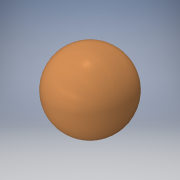
# Autodesk Inventor part: Ball
Saved by Autodesk Inventor 2016 (Build 200138000, 138)
## iProperties
Created: 2016-01-18
Part Number: Ball
Material: Polyurethane Foam
Document SubType Name: Modeling
Designer: yash
Density: 0.032 g/cm^3
Appearance: Coarse Textured - Umber
Author: yash
Autodesk Inventor part; units mm, degrees
ref_plane "YZ Plane" through (0, 0, 0) normal (1, 0, 0) x (0, 1, 0)
ref_plane "XZ Plane" through (0, 0, 0) normal (0, 1, 0) x (-1, 0, 0)
ref_plane "XY Plane" through (0, 0, 0) normal (0, 0, 1) x (1, 0, 0)
sketch "Sketch1" plane through (0, 0, 0) normal (0, 1, 0) x (-1, 0, 0)
  circle A0 centre (0, 0) radius 101.6
  line L0 (0, -101.6) -> (0, 101.6)
  dimension "d0" = 203.2
  dimension "d1" = 0
  constraints: 2 end point, 2 point on circle, 1 centre point, 1 coincident, 1 vertical
  measures "d0" diameter of A0
  measures "d1" distance from line of point (0, 0) L0
revolve "Revolution1" add sketch "Sketch1" angle 360 about axis through (0, 0, -101.6) along (0, 0, 1)
body "Solid1"
